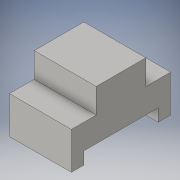
# Autodesk Inventor part: Unit 7.1 part 2
Saved by Autodesk Inventor 2016 (Build 200138000, 138)
## iProperties
Created: 2017-03-02
Part Number: Unit 7.1 part 2
Material: Generic
Document SubType Name: Modeling
Designer: 196918
Density: 1 g/cm^3
Appearance: Default
Author: 196918
Autodesk Inventor part; units mm, degrees
ref_plane "YZ Plane" through (0, 0, 0) normal (1, 0, 0) x (0, 1, 0)
ref_plane "XZ Plane" through (0, 0, 0) normal (0, 1, 0) x (-1, 0, 0)
ref_plane "XY Plane" through (0, 0, 0) normal (0, 0, 1) x (1, 0, 0)
sketch "Sketch1" plane through (0, 0, 0) normal (0, 1, 0) x (-1, 0, 0)
  line L0 (-12.1689, 29.6355) -> (-43.9189, 29.6355)
  line L1 (-43.9189, 29.6355) -> (-43.9189, -21.1645)
  line L2 (-43.9189, -21.1645) -> (-12.1689, -21.1645)
  line L3 (-12.1689, -21.1645) -> (-12.1689, 29.6355)
  point P0 (0, 0)
  dimension "d0" = 31.75
  dimension "d1" = 50.8
  constraints: 8 end point, 2 parallel, 1 horizontal, 1 perpendicular
  measures "d0" distance of L2.end L1.end
  measures "d1" distance of L1.end L0.end
extrude "Extrusion1" add sketch "Sketch1" along normal blind 12.7
sketch "Sketch2" plane through (0, 12.7, 0) normal (0, 1, 0) x (1, 0, 0)
  line L0 (43.9189, -29.6355) -> (43.9189, 21.1645) projected
  line L1 (43.9189, 21.1645) -> (43.9189, 8.4645)
  line L2 (43.9189, -29.6355) -> (43.9189, -16.9355)
  line L3 (12.1689, 21.1645) -> (12.1689, -29.6355) projected
  line L4 (43.9189, -16.9355) -> (12.1689, -16.9355)
  line L5 (12.1689, -16.9355) -> (12.1689, 8.4645)
  line L6 (12.1689, 8.4645) -> (43.9189, 8.4645)
  line L7 (43.9189, 8.4645) -> (43.9189, -16.9355)
  point P0 (0, 0)
  dimension "d4" = 12.7
  dimension "d5" = 12.7
  constraints: 12 end point, 3 point on line, 2 parallel, 1 horizontal, 1 perpendicular
  measures "d4" distance of L0.end L1.end
  measures "d5" distance of L0.start L2.end
extrude "Extrusion2" add sketch "Sketch2" along normal blind 12.7
sketch "Sketch3" plane through (0, 0, 0) normal (0, -1, 0) x (1, 0, 0)
  line L0 (43.9189, -21.1645) -> (12.1689, -21.1645) projected
  line L1 (12.1689, -21.1645) -> (12.1689, -8.4645) projected
  line L2 (43.9189, -21.1645) -> (12.1689, -21.1645)
  line L3 (12.1689, -21.1645) -> (12.1689, -14.8145)
  line L4 (12.1689, -14.8145) -> (43.9189, -14.8145)
  line L5 (43.9189, -14.8145) -> (43.9189, -21.1645)
  line L6 (43.9189, 29.6355) -> (43.9189, 16.9355) projected
  line L7 (43.9189, 29.6355) -> (12.1689, 29.6355)
  line L8 (12.1689, 29.6355) -> (12.1689, 23.2855)
  line L9 (12.1689, 23.2855) -> (43.9189, 23.2855)
  line L10 (43.9189, 23.2855) -> (43.9189, 29.6355)
  point P0 (0, 0)
  dimension "d8" = 6.35
  dimension "d9" = 6.35
  constraints: 16 end point, 4 parallel, 2 horizontal, 2 perpendicular, 1 midpoint, 1 point on line
  measures "d8" distance of L2.end L3.end
  measures "d9" distance of L8.end L7.end
extrude "Extrusion3" add sketch "Sketch3" along normal blind 6.35
body "Solid1"
